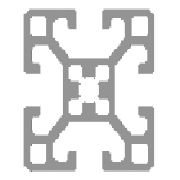
# Autodesk Inventor part: 10-540
Saved by Autodesk Inventor 2022 (Build 260153000, 153)
## iProperties
Created: 2021-12-28
Part Number: 10-540
Material: Generico
Document SubType Name: Modeling
Designer: matte
Standards Organization: 40 series
Language: it-IT
Size Designation: 10-540
Categories: <MemberInstance><Categories><Category DisplayName="Forme strutturali" InternalName="089c4875-fa83-4c05-b084-43b9cc11f5ed" Mnemonic="GRDR"><CategoryParameter DisplayName="Massa per unità di lunghezza" InternalName="0bb95a10-148f-4027-a459-38d7b056702a" Mnemonic="shpmass"/><CategoryParameter DisplayName="Area sezione" InternalName="1ff91680-64b0-4202-b9a3-7fd3f94bba3b" Mnemonic="secarea"/><CategoryParameter DisplayName="Raggio di girazione (x)" InternalName="25778675-03e9-40c1-b6a8-4a9ed693320d" Mnemonic="gyrradx"/><CategoryParameter DisplayName="Modulo di rigidità torsionale" InternalName="26c1ec35-5026-4c63-ad0a-751cf684a536" Mnemonic="torrigmod"/><CategoryParameter DisplayName="Distanza del baricentro X-X" InternalName="26c9bdb8-9c79-4b4f-a92e-8e197583c9c4" Mnemonic="grcendistX"/><CategoryParameter DisplayName="ID membro precedente" InternalName="340afe4f-75d7-48d3-ab7d-943f3c3da468" Mnemonic="LegacyMemberID"/><CategoryParameter DisplayName="Lunghezza base" InternalName="42e34263-8f20-4d0e-ad48-bf1385b87c24" Mnemonic="shplen"/><CategoryParameter DisplayName="Momento di inerzia (y)" InternalName="4b9f58ea-bced-460e-81ea-3d29ca5a49e3" Mnemonic="inermomy"/><CategoryParameter DisplayName="Momento di inerzia (x)" InternalName="4cd780bc-73d7-43ac-917a-579e5cbd684d" Mnemonic="inermomx"/><CategoryParameter DisplayName="Punto di base personalizzato" InternalName="4f1d1b73-316d-484b-a3df-9cbabb16eb77" Mnemonic="shpBasePoint"/><CategoryParameter DisplayName="Altezza forma" InternalName="50274e7d-5ac0-4796-92cb-c59e54983c67" Mnemonic="shpheig"/><CategoryParameter DisplayName="Modulo sezione (y)" InternalName="59eaa5e9-d227-48dc-b6c1-6920f96e0f95" Mnemonic="secmody"/><CategoryParameter DisplayName="Designazione sezione" InternalName="5a64d034-428d-49c8-ba32-7619764de20f" Mnemonic="shpdes"/><CategoryParameter DisplayName="Modulo sezione (x)" InternalName="72cfad18-cf51-4ed4-aaa7-c6b224f8419f" Mnemonic="secmodx"/><CategoryParameter DisplayName="Modulo di sezione torsionale" InternalName="7c55a8dc-8844-49f9-a867-cc677b30ec9a" Mnemonic="torsecmod"/><CategoryParameter DisplayName="Larghezza forma" InternalName="7c717d54-a18f-4666-b4d4-573cce22c62c" Mnemonic="shpwdth"/><CategoryParameter DisplayName="Spessore seconda forma" InternalName="9251a8e1-85fd-4e47-af99-afdb762317d9" Mnemonic="shpthick2"/><CategoryParameter DisplayName="Guarnizione piatta creata" InternalName="9c666724-f362-4ea7-ac62-f6a007de5c69" Mnemonic="shpFGAuto"/><CategoryParameter DisplayName="Distanza del baricentro Y-Y" InternalName="bcc4fb17-7af4-436a-8f8c-d0aa3b0248c5" Mnemonic="grcendistY"/><CategoryParameter DisplayName="Raggio di girazione (y)" InternalName="bfa18ebe-1636-4dbe-8d42-b263e0b73184" Mnemonic="gyrrady"/><CategoryParameter DisplayName="Spessore forma" InternalName="d109cf76-8eb4-42fc-9800-4409734adc67" Mnemonic="shpthick"/><CategoryParameter DisplayName="Coefficiente di spostamento taglio" InternalName="de4c90c6-aaa8-468f-a335-6737b311b5d3" Mnemonic="shdispc"/><Category DisplayName="Altro" InternalName="f02205ff-2390-476f-921c-0b3185f88e84" Mnemonic="OTHSHP"><CategoryParameter DisplayName="Momento di inerzia (y)" InternalName="044c654e-f649-48ac-84cc-650a29ae31ca" Mnemonic="inermomy"/><CategoryParameter DisplayName="Spessore forma" InternalName="12b1a788-9233-48fd-a933-2df8ff42b15f" Mnemonic="shpthick"/><CategoryParameter DisplayName="Massa per unità di lunghezza" InternalName="2fd289d6-9394-4d2d-97e6-6659d7d4551d" Mnemonic="shpmass"/><CategoryParameter DisplayName="Raggio di girazione (y)" InternalName="743e1dfe-1bba-408b-b985-cf752b207386" Mnemonic="gyrrady"/><CategoryParameter DisplayName="Modulo sezione (y)" InternalName="88b8bff9-a616-4028-93d5-ed4f79680d13" Mnemonic="secmody"/><CategoryParameter DisplayName="Area sezione" InternalName="c46ecdf8-b6eb-4db9-8b25-30258930c1e3" Mnemonic="secarea"/><CategoryParameter DisplayName="Modulo sezione (x)" InternalName="cac70804-9d39-43bb-be17-56ea1f39a6c2" Mnemonic="secmodx"/><CategoryParameter DisplayName="Momento di inerzia (x)" InternalName="ec6737bc-264f-43ed-b0bd-f6d410c2718d" Mnemonic="inermomx"/><CategoryParameter DisplayName="Raggio di girazione (x)" InternalName="ee72c61e-565e-4fd6-b448-66e1e1abcb7e" Mnemonic="gyrradx"/></Category></Category><Category DisplayName="TipoDati" InternalName="23b78d0f-2648-40c6-8793-ca6db495c9e8" Mnemonic="DATATYPE"><CategoryParameter DisplayName="NomeVisualizzazione" InternalName="05415f3d-3907-474b-a020-eb9d644f4cf3" Mnemonic="DISPLAYNAME"/><CategoryParameter DisplayName="Norme" InternalName="0c0a119c-1e12-4c84-803f-101930972f5e" Mnemonic="STANDARD"/><CategoryParameter DisplayName="Descrizione" InternalName="13903e3d-64b1-4950-80da-f627842ea37f" Mnemonic="DESCRIPTION"/><CategoryParameter DisplayName="Designazione" InternalName="2675968c-4ce5-49e0-a4f5-552d29089031" Mnemonic="DESIGNATION"/><CategoryParameter DisplayName="Riga di default" InternalName="2af9ec52-faaa-4026-b378-f9fa4afca842" Mnemonic="DEFAULTROW"/><CategoryParameter DisplayName="Nome cartella" InternalName="3f06958e-8713-4116-9be7-ed6184ecc97b" Mnemonic="FOLDERNAME"/><CategoryParameter DisplayName="Guid revisione" InternalName="45a75005-10b1-4dfc-8d6d-dfe629f0b93c" Mnemonic="REVISIONGUID"/><CategoryParameter DisplayName="NomeFile" InternalName="8b46a4cc-9585-4fed-90c3-899f57e09a73" Mnemonic="FILENAME"/><CategoryParameter DisplayName="SocietàNorme" InternalName="8f5914e1-4693-403f-8ab5-d37768198c9d" Mnemonic="STDSORG"/><CategoryParameter DisplayName="Versione famiglia" InternalName="914462f6-6e19-4b14-ba84-155b9680b1d0" Mnemonic="FAMILYREVISION"/><CategoryParameter DisplayName="Revisione norme" InternalName="91d5a463-65c2-4fde-b823-3b7fea5e8e17" Mnemonic="STANDARDREVISION"/><CategoryParameter DisplayName="Revisione membro" InternalName="a65d44b9-392f-4f4f-857b-e4b3d54996fe" Mnemonic="MEMBERREVISION"/><CategoryParameter DisplayName="FormatoPianoRitaglio" InternalName="bc51e27b-3422-4e78-93ef-cec197ddf230" Mnemonic="CLIPFORMAT"/><CategoryParameter DisplayName="Produttore" InternalName="cd6c7a72-a28a-4e50-99a9-2c7f4e13e5ad" Mnemonic="MANUFACTURER"/><CategoryParameter DisplayName="NomeInterno" InternalName="cf1d0246-76d9-4b4a-8305-fa0409afb5c1" Mnemonic="INTERNALNAME"/><CategoryParameter DisplayName="Èmetrico" InternalName="e2385c5b-1ea4-4823-96a8-8de651266ec3" Mnemonic="ISMETRIC"/><Category DisplayName="Parte" InternalName="c0e0b642-3bcb-4cc8-9e80-f96d35c4afa4" Mnemonic="PART"><CategoryParameter DisplayName="Numero parte" InternalName="016b6077-bfbe-49bd-92c9-d8d59c39c941" Mnemonic="PARTNUMBER"/><CategoryParameter DisplayName="Numero di magazzino" InternalName="4dba7c1c-e26c-444e-836c-b08b433409a8" Mnemonic="STOCKNUMBER"/><CategoryParameter DisplayName="Chiave materiale" InternalName="5c9a8adb-dd2b-4535-b97f-0a94a95fe41f" Mnemonic="MATERIALKEY"/><CategoryParameter DisplayName="Materiale" InternalName="818a152a-d3c3-49ca-80ee-df7d91421b8e" Mnemonic="MATERIAL"/></Category></Category></Categories><FamilyTemplate Id="10-540"><FamilyTemplateParameters><FamilyTemplateParameter ObjectType="kModelParameterObject" ValueType="xs:double" Id="12" ObjectReferenceKey="d0"/><FamilyTemplateParameter ObjectType="kPartComponentDefinitionObject" ValueType="xs:string" Id="23" SubObjectId="Material"/><FamilyTemplateParameter ObjectType="kPropertyObject" ValueType="xs:string" Id="26" ObjectReferenceKey="{32853F0F-3444-11d1-9E93-0060B03C1CA6}" SubObjectId="5"/><FamilyTemplateParameter ObjectType="kPropertyObject" ValueType="xs:string" Id="27" ObjectReferenceKey="{32853F0F-3444-11d1-9E93-0060B03C1CA6}" SubObjectId="52"/></FamilyTemplateParameters></FamilyTemplate><CategoryParameterMap><ParamToTemplateMap><ParamToTemplate CategoryParameter="//CategoryParameter[@InternalName='cf1d0246-76d9-4b4a-8305-fa0409afb5c1']" ConstantValue="7d6ce073-411f-4b6a-829f-d390fd53fc07"/><ParamToTemplate CategoryParameter="//CategoryParameter[@InternalName='45a75005-10b1-4dfc-8d6d-dfe629f0b93c']" ConstantValue="1b59e780-9fa2-4ac4-888e-f8f724c6c2fd"/><ParamToTemplate CategoryParameter="//CategoryParameter[@InternalName='3f06958e-8713-4116-9be7-ed6184ecc97b']" ConstantValue="10-540"/><ParamToTemplate CategoryParameter="//CategoryParameter[@InternalName='8f5914e1-4693-403f-8ab5-d37768198c9d']" ConstantValue="40 series"/><ParamToTemplate CategoryParameter="//CategoryParameter[@InternalName='0c0a119c-1e12-4c84-803f-101930972f5e']" TemplateParameter="18"/><ParamToTemplate CategoryParameter="//CategoryParameter[@InternalName='91d5a463-65c2-4fde-b823-3b7fea5e8e17']" TemplateParameter="19"/><ParamToTemplate CategoryParameter="//CategoryParameter[@InternalName='cd6c7a72-a28a-4e50-99a9-2c7f4e13e5ad']" TemplateParameter="20"/><ParamToTemplate CategoryParameter="//CategoryParameter[@InternalName='13903e3d-64b1-4950-80da-f627842ea37f']" TemplateParameter="22"/><ParamToTemplate CategoryParameter="//CategoryParameter[@InternalName='05415f3d-3907-474b-a020-eb9d644f4cf3']" ConstantValue="10-540"/><ParamToTemplate CategoryParameter="//CategoryParameter[@InternalName='914462f6-6e19-4b14-ba84-155b9680b1d0']" ConstantValue="11"/><ParamToTemplate CategoryParameter="//CategoryParameter[@InternalName='bc51e27b-3422-4e78-93ef-cec197ddf230']" ConstantValue="CF_INVENTOR.STDPARTS"/><ParamToTemplate CategoryParameter="//CategoryParameter[@InternalName='e2385c5b-1ea4-4823-96a8-8de651266ec3']" ConstantValue="true"/><ParamToTemplate CategoryParameter="//CategoryParameter[@InternalName='2af9ec52-faaa-4026-b378-f9fa4afca842']" ConstantValue="1"/><ParamToTemplate CategoryParameter="//CategoryParameter[@InternalName='9c666724-f362-4ea7-ac62-f6a007de5c69']" ConstantValue="1"/><ParamToTemplate CategoryParameter="//CategoryParameter[@InternalName='8b46a4cc-9585-4fed-90c3-899f57e09a73']" ConstantValue="10-540"/><ParamToTemplate CategoryParameter="//CategoryParameter[@InternalName='a65d44b9-392f-4f4f-857b-e4b3d54996fe']" ConstantValue="cf6cafbf-75ec-4cf3-9738-ab9345264871"/><ParamToTemplate CategoryParameter="//CategoryParameter[@InternalName='a65d44b9-392f-4f4f-857b-e4b3d54996fe']" ConstantValue="cf6cafbf-75ec-4cf3-9738-ab9345264871"/><ParamToTemplate CategoryParameter="//CategoryParameter[@InternalName='2675968c-4ce5-49e0-a4f5-552d29089031']" TemplateParameter="27"/><ParamToTemplate CategoryParameter="//CategoryParameter[@InternalName='818a152a-d3c3-49ca-80ee-df7d91421b8e']" TemplateParameter="23"/><ParamToTemplate CategoryParameter="//CategoryParameter[@InternalName='016b6077-bfbe-49bd-92c9-d8d59c39c941']" TemplateParameter="26"/><ParamToTemplate CategoryParameter="//CategoryParameter[@InternalName='42e34263-8f20-4d0e-ad48-bf1385b87c24']" TemplateParameter="12"/></ParamToTemplateMap></CategoryParameterMap></MemberInstance>
Density: 1 g/cm^3
Appearance: Default
IsCustomPart: 1
Author: matte
MXEDIT: true
G_L: 100.000 mm
Autodesk Inventor part; units mm, degrees
ref_plane "YZ Plane" through (0, 0, 0) normal (1, 0, 0) x (0, 1, 0)
ref_plane "XY Plane" through (0, 0, 0) normal (0, 0, 1) x (1, 0, 0)
ref_plane "Start Plane" through (0, 0, 0) normal (0, 1, 0) x (-1, 0, 0)
ref_plane "End Plane" through (0, 100, 0) normal (0, 1, 0) x (-1, 0, 0)
sketch "Sketch1" plane through (0, 0, 0) normal (0, 1, 0) x (-1, 0, 0)
  arc A0 (-2.032, 3.5877) -> (-1.3254, 3.1202) centre (-1.524, 3.5877) ccw
  arc A1 (1.3254, 3.1202) -> (-1.3254, 3.1202) centre (0, 0) ccw
  arc A2 (1.3254, 3.1202) -> (2.032, 3.5877) centre (1.524, 3.5877) ccw
  line L0 (2.032, 3.5877) -> (2.032, 5.522)
  arc A3 (2.794, 6.284) -> (2.032, 5.522) centre (2.794, 5.522) ccw
  line L1 (2.794, 6.284) -> (5.522, 6.284)
  arc A4 (6.284, 5.522) -> (5.522, 6.284) centre (5.522, 5.522) ccw
  line L2 (6.284, 5.522) -> (6.284, 2.794)
  arc A5 (5.522, 2.032) -> (6.284, 2.794) centre (5.522, 2.794) ccw
  line L3 (5.522, 2.032) -> (3.5877, 2.032)
  arc A6 (3.5877, 2.032) -> (3.1202, 1.3254) centre (3.5877, 1.524) ccw
  arc A7 (3.1202, -1.3254) -> (3.1202, 1.3254) centre (0, 0) ccw
  arc A8 (3.1202, -1.3254) -> (3.5877, -2.032) centre (3.5877, -1.524) ccw
  line L4 (3.5877, -2.032) -> (5.522, -2.032)
  arc A9 (6.284, -2.794) -> (5.522, -2.032) centre (5.522, -2.794) ccw
  line L5 (6.284, -2.794) -> (6.284, -5.522)
  arc A10 (5.522, -6.284) -> (6.284, -5.522) centre (5.522, -5.522) ccw
  line L6 (5.522, -6.284) -> (2.794, -6.284)
  arc A11 (2.032, -5.522) -> (2.794, -6.284) centre (2.794, -5.522) ccw
  line L7 (2.032, -5.522) -> (2.032, -3.5877)
  arc A12 (2.032, -3.5877) -> (1.3254, -3.1202) centre (1.524, -3.5877) ccw
  arc A13 (-1.3254, -3.1202) -> (1.3254, -3.1202) centre (0, 0) ccw
  arc A14 (-1.3254, -3.1202) -> (-2.032, -3.5877) centre (-1.524, -3.5877) ccw
  line L8 (-2.032, -3.5877) -> (-2.032, -5.522)
  arc A15 (-2.794, -6.284) -> (-2.032, -5.522) centre (-2.794, -5.522) ccw
  line L9 (-2.794, -6.284) -> (-5.522, -6.284)
  arc A16 (-6.284, -5.522) -> (-5.522, -6.284) centre (-5.522, -5.522) ccw
  line L10 (-6.284, -5.522) -> (-6.284, -2.794)
  arc A17 (-5.522, -2.032) -> (-6.284, -2.794) centre (-5.522, -2.794) ccw
  line L11 (-5.522, -2.032) -> (-3.5877, -2.032)
  arc A18 (-3.5877, -2.032) -> (-3.1202, -1.3254) centre (-3.5877, -1.524) ccw
  arc A19 (-3.1202, 1.3254) -> (-3.1202, -1.3254) centre (0, 0) ccw
  arc A20 (-3.1202, 1.3254) -> (-3.5877, 2.032) centre (-3.5877, 1.524) ccw
  line L12 (-3.5877, 2.032) -> (-5.522, 2.032)
  arc A21 (-6.284, 2.794) -> (-5.522, 2.032) centre (-5.522, 2.794) ccw
  line L13 (-6.284, 2.794) -> (-6.284, 5.522)
  arc A22 (-5.522, 6.284) -> (-6.284, 5.522) centre (-5.522, 5.522) ccw
  line L14 (-5.522, 6.284) -> (-2.794, 6.284)
  arc A23 (-2.032, 5.522) -> (-2.794, 6.284) centre (-2.794, 5.522) ccw
  line L15 (-2.032, 5.522) -> (-2.032, 3.5877)
  line L16 (18.4252, 17.1552) -> (18.4252, 14.1732)
  arc A24 (17.1552, 12.9032) -> (18.4252, 14.1732) centre (17.1552, 14.1732) ccw
  line L17 (17.1552, 12.9032) -> (14.1732, 12.9032)
  arc A25 (12.9032, 14.1732) -> (14.1732, 12.9032) centre (14.1732, 14.1732) ccw
  line L18 (12.9032, 14.1732) -> (12.9032, 17.1552)
  arc A26 (14.1732, 18.4252) -> (12.9032, 17.1552) centre (14.1732, 17.1552) ccw
  line L19 (14.1732, 18.4252) -> (17.1552, 18.4252)
  arc A27 (18.4252, 17.1552) -> (17.1552, 18.4252) centre (17.1552, 17.1552) ccw
  line L20 (17.1552, -18.4252) -> (14.1732, -18.4252)
  arc A28 (12.9032, -17.1552) -> (14.1732, -18.4252) centre (14.1732, -17.1552) ccw
  line L21 (12.9032, -17.1552) -> (12.9032, -14.1732)
  arc A29 (14.1732, -12.9032) -> (12.9032, -14.1732) centre (14.1732, -14.1732) ccw
  line L22 (14.1732, -12.9032) -> (17.1552, -12.9032)
  arc A30 (18.4252, -14.1732) -> (17.1552, -12.9032) centre (17.1552, -14.1732) ccw
  line L23 (18.4252, -14.1732) -> (18.4252, -17.1552)
  arc A31 (17.1552, -18.4252) -> (18.4252, -17.1552) centre (17.1552, -17.1552) ccw
  line L24 (-18.4252, -17.1552) -> (-18.4252, -14.1732)
  arc A32 (-17.1552, -12.9032) -> (-18.4252, -14.1732) centre (-17.1552, -14.1732) ccw
  line L25 (-17.1552, -12.9032) -> (-14.1732, -12.9032)
  arc A33 (-12.9032, -14.1732) -> (-14.1732, -12.9032) centre (-14.1732, -14.1732) ccw
  line L26 (-12.9032, -14.1732) -> (-12.9032, -17.1552)
  arc A34 (-14.1732, -18.4252) -> (-12.9032, -17.1552) centre (-14.1732, -17.1552) ccw
  line L27 (-14.1732, -18.4252) -> (-17.1552, -18.4252)
  arc A35 (-18.4252, -17.1552) -> (-17.1552, -18.4252) centre (-17.1552, -17.1552) ccw
  line L28 (-14.1732, 12.9032) -> (-17.1552, 12.9032)
  arc A36 (-18.4252, 14.1732) -> (-17.1552, 12.9032) centre (-17.1552, 14.1732) ccw
  line L29 (-18.4252, 14.1732) -> (-18.4252, 17.1552)
  arc A37 (-17.1552, 18.4252) -> (-18.4252, 17.1552) centre (-17.1552, 17.1552) ccw
  line L30 (-17.1552, 18.4252) -> (-14.1732, 18.4252)
  arc A38 (-12.9032, 17.1552) -> (-14.1732, 18.4252) centre (-14.1732, 17.1552) ccw
  line L31 (-12.9032, 17.1552) -> (-12.9032, 14.1732)
  arc A39 (-14.1732, 12.9032) -> (-12.9032, 14.1732) centre (-14.1732, 14.1732) ccw
  arc A40 (20, 17) -> (17, 20) centre (17, 17) ccw
  line L32 (4.1, 18.5014) -> (4.1, 16.0122)
  arc A41 (4.1, 16.0122) -> (4.608, 15.5042) centre (4.608, 16.0122) ccw
  line L33 (4.608, 15.5042) -> (5.8018, 15.5042)
  arc A42 (5.8018, 15.5042) -> (6.3098, 16.0122) centre (5.8018, 16.0122) ccw
  line L34 (6.3098, 16.0122) -> (6.3098, 17.2822)
  arc A43 (6.8178, 17.7902) -> (6.3098, 17.2822) centre (6.8178, 17.2822) ccw
  line L35 (6.8178, 17.7902) -> (9.9314, 17.7902)
  arc A44 (11.43, 16.2916) -> (9.9314, 17.7902) centre (9.9314, 16.2916) ccw
  line L36 (11.43, 16.2916) -> (11.43, 13.6133)
  arc A45 (10.9911, 12.5536) -> (11.43, 13.6133) centre (9.9314, 13.6133) ccw
  line L37 (10.9911, 12.5536) -> (6.6336, 8.1961)
  arc A46 (5.5739, 7.7572) -> (6.6336, 8.1961) centre (5.5739, 9.2558) ccw
  line L38 (5.5739, 7.7572) -> (-5.5739, 7.7572)
  arc A47 (-6.6336, 8.1961) -> (-5.5739, 7.7572) centre (-5.5739, 9.2558) ccw
  line L39 (-6.6336, 8.1961) -> (-10.9911, 12.5536)
  arc A48 (-11.43, 13.6133) -> (-10.9911, 12.5536) centre (-9.9314, 13.6133) ccw
  line L40 (-11.43, 13.6133) -> (-11.43, 16.2916)
  arc A49 (-9.9314, 17.7902) -> (-11.43, 16.2916) centre (-9.9314, 16.2916) ccw
  line L41 (-9.9314, 17.7902) -> (-6.8178, 17.7902)
  arc A50 (-6.3098, 17.2822) -> (-6.8178, 17.7902) centre (-6.8178, 17.2822) ccw
  line L42 (-6.3098, 17.2822) -> (-6.3098, 16.0122)
  arc A51 (-6.3098, 16.0122) -> (-5.8018, 15.5042) centre (-5.8018, 16.0122) ccw
  line L43 (-5.8018, 15.5042) -> (-4.608, 15.5042)
  arc A52 (-4.608, 15.5042) -> (-4.1, 16.0122) centre (-4.608, 16.0122) ccw
  line L44 (-4.1, 16.0122) -> (-4.1, 18.5014)
  line L45 (-15.5702, 20) -> (-17, 20)
  arc A53 (-17, 20) -> (-20, 17) centre (-17, 17) ccw
  line L46 (-20, 17) -> (-20, 15.5702)
  line L47 (-18.5014, 4.1) -> (-16.0122, 4.1)
  arc A54 (-16.0122, 4.1) -> (-15.5042, 4.608) centre (-16.0122, 4.608) ccw
  line L48 (-15.5042, 4.608) -> (-15.5042, 5.8018)
  arc A55 (-15.5042, 5.8018) -> (-16.0122, 6.3098) centre (-16.0122, 5.8018) ccw
  line L49 (-16.0122, 6.3098) -> (-17.2822, 6.3098)
  arc A56 (-17.7902, 6.8178) -> (-17.2822, 6.3098) centre (-17.2822, 6.8178) ccw
  line L50 (-17.7902, 6.8178) -> (-17.7902, 9.9314)
  arc A57 (-16.2916, 11.43) -> (-17.7902, 9.9314) centre (-16.2916, 9.9314) ccw
  line L51 (-16.2916, 11.43) -> (-13.6133, 11.43)
  arc A58 (-12.5536, 10.9911) -> (-13.6133, 11.43) centre (-13.6133, 9.9314) ccw
  line L52 (-12.5536, 10.9911) -> (-8.1961, 6.6336)
  arc A59 (-7.7572, 5.5739) -> (-8.1961, 6.6336) centre (-9.2558, 5.5739) ccw
  line L53 (-7.7572, 5.5739) -> (-7.7572, -5.5739)
  arc A60 (-8.1961, -6.6336) -> (-7.7572, -5.5739) centre (-9.2558, -5.5739) ccw
  line L54 (-8.1961, -6.6336) -> (-12.5536, -10.9911)
  arc A61 (-13.6133, -11.43) -> (-12.5536, -10.9911) centre (-13.6133, -9.9314) ccw
  line L55 (-13.6133, -11.43) -> (-16.2916, -11.43)
  arc A62 (-17.7902, -9.9314) -> (-16.2916, -11.43) centre (-16.2916, -9.9314) ccw
  line L56 (-17.7902, -9.9314) -> (-17.7902, -6.8178)
  arc A63 (-17.2822, -6.3098) -> (-17.7902, -6.8178) centre (-17.2822, -6.8178) ccw
  line L57 (-17.2822, -6.3098) -> (-16.0122, -6.3098)
  arc A64 (-16.0122, -6.3098) -> (-15.5042, -5.8018) centre (-16.0122, -5.8018) ccw
  line L58 (-15.5042, -5.8018) -> (-15.5042, -4.608)
  arc A65 (-15.5042, -4.608) -> (-16.0122, -4.1) centre (-16.0122, -4.608) ccw
  line L59 (-16.0122, -4.1) -> (-18.5014, -4.1)
  arc A66 (-18.5014, -4.1) -> (-20, -5.5986) centre (-18.5014, -5.5986) ccw
  arc A67 (-20, -17) -> (-17, -20) centre (-17, -17) ccw
  line L60 (-4.1, -18.5014) -> (-4.1, -16.0122)
  arc A68 (-5.5986, -20) -> (-4.1, -18.5014) centre (-5.5986, -18.5014) ccw
  arc A69 (-4.1, -16.0122) -> (-4.608, -15.5042) centre (-4.608, -16.0122) ccw
  line L61 (-4.608, -15.5042) -> (-5.8018, -15.5042)
  arc A70 (-5.8018, -15.5042) -> (-6.3098, -16.0122) centre (-5.8018, -16.0122) ccw
  line L62 (-6.3098, -16.0122) -> (-6.3098, -17.2822)
  arc A71 (-6.8178, -17.7902) -> (-6.3098, -17.2822) centre (-6.8178, -17.2822) ccw
  line L63 (-6.8178, -17.7902) -> (-9.9314, -17.7902)
  arc A72 (-11.43, -16.2916) -> (-9.9314, -17.7902) centre (-9.9314, -16.2916) ccw
  line L64 (-11.43, -16.2916) -> (-11.43, -13.6133)
  arc A73 (-10.9911, -12.5536) -> (-11.43, -13.6133) centre (-9.9314, -13.6133) ccw
  line L65 (-10.9911, -12.5536) -> (-6.6336, -8.1961)
  arc A74 (-5.5739, -7.7572) -> (-6.6336, -8.1961) centre (-5.5739, -9.2558) ccw
  line L66 (-5.5739, -7.7572) -> (5.5739, -7.7572)
  arc A75 (6.6336, -8.1961) -> (5.5739, -7.7572) centre (5.5739, -9.2558) ccw
  line L67 (6.6336, -8.1961) -> (10.9911, -12.5536)
  arc A76 (11.43, -13.6133) -> (10.9911, -12.5536) centre (9.9314, -13.6133) ccw
  line L68 (11.43, -13.6133) -> (11.43, -16.2916)
  arc A77 (9.9314, -17.7902) -> (11.43, -16.2916) centre (9.9314, -16.2916) ccw
  line L69 (9.9314, -17.7902) -> (6.8178, -17.7902)
  arc A78 (6.3098, -17.2822) -> (6.8178, -17.7902) centre (6.8178, -17.2822) ccw
  line L70 (6.3098, -17.2822) -> (6.3098, -16.0122)
  arc A79 (6.3098, -16.0122) -> (5.8018, -15.5042) centre (5.8018, -16.0122) ccw
  line L71 (5.8018, -15.5042) -> (4.608, -15.5042)
  arc A80 (4.608, -15.5042) -> (4.1, -16.0122) centre (4.608, -16.0122) ccw
  line L72 (4.1, -16.0122) -> (4.1, -18.5014)
  arc A81 (4.1, -18.5014) -> (5.5986, -20) centre (5.5986, -18.5014) ccw
  arc A82 (17, -20) -> (20, -17) centre (17, -17) ccw
  line L73 (18.5014, -4.1) -> (16.0122, -4.1)
  arc A83 (20, -5.5986) -> (18.5014, -4.1) centre (18.5014, -5.5986) ccw
  arc A84 (16.0122, -4.1) -> (15.5042, -4.608) centre (16.0122, -4.608) ccw
  line L74 (15.5042, -4.608) -> (15.5042, -5.8018)
  arc A85 (15.5042, -5.8018) -> (16.0122, -6.3098) centre (16.0122, -5.8018) ccw
  line L75 (16.0122, -6.3098) -> (17.2822, -6.3098)
  arc A86 (17.7902, -6.8178) -> (17.2822, -6.3098) centre (17.2822, -6.8178) ccw
  line L76 (17.7902, -6.8178) -> (17.7902, -9.9314)
  arc A87 (16.2916, -11.43) -> (17.7902, -9.9314) centre (16.2916, -9.9314) ccw
  line L77 (16.2916, -11.43) -> (13.6133, -11.43)
  arc A88 (12.5536, -10.9911) -> (13.6133, -11.43) centre (13.6133, -9.9314) ccw
  line L78 (12.5536, -10.9911) -> (8.1961, -6.6336)
  arc A89 (7.7572, -5.5739) -> (8.1961, -6.6336) centre (9.2558, -5.5739) ccw
  line L79 (7.7572, -5.5739) -> (7.7572, 5.5739)
  arc A90 (8.1961, 6.6336) -> (7.7572, 5.5739) centre (9.2558, 5.5739) ccw
  line L80 (8.1961, 6.6336) -> (12.5536, 10.9911)
  arc A91 (13.6133, 11.43) -> (12.5536, 10.9911) centre (13.6133, 9.9314) ccw
  line L81 (13.6133, 11.43) -> (16.2916, 11.43)
  arc A92 (17.7902, 9.9314) -> (16.2916, 11.43) centre (16.2916, 9.9314) ccw
  line L82 (17.7902, 9.9314) -> (17.7902, 6.8178)
  arc A93 (17.2822, 6.3098) -> (17.7902, 6.8178) centre (17.2822, 6.8178) ccw
  line L83 (17.2822, 6.3098) -> (16.0122, 6.3098)
  arc A94 (16.0122, 6.3098) -> (15.5042, 5.8018) centre (16.0122, 5.8018) ccw
  line L84 (15.5042, 5.8018) -> (15.5042, 4.608)
  arc A95 (15.5042, 4.608) -> (16.0122, 4.1) centre (16.0122, 4.608) ccw
  line L85 (16.0122, 4.1) -> (18.5014, 4.1)
  line L86 (-15.5702, 20) -> (-5.5986, 20)
  arc A96 (-4.1, 18.5014) -> (-5.5986, 20) centre (-5.5986, 18.5014) ccw
  line L87 (-20, 15.5702) -> (-20, 5.5986)
  arc A97 (-20, 5.5986) -> (-18.5014, 4.1) centre (-18.5014, 5.5986) ccw
  line L88 (17, 20) -> (5.5986, 20)
  arc A98 (5.5986, 20) -> (4.1, 18.5014) centre (5.5986, 18.5014) ccw
  line L89 (20, 17) -> (20, 5.5986)
  arc A99 (18.5014, 4.1) -> (20, 5.5986) centre (18.5014, 5.5986) ccw
  line L90 (20, -17) -> (20, -5.5986)
  line L91 (17, -20) -> (5.5986, -20)
  line L92 (-17, -20) -> (-5.5986, -20)
  line L93 (-20, -17) -> (-20, -5.5986)
  constraints: 200 point on circle, 188 end point, 100 centre point, 43 horizontal, 43 vertical, 403 other
extrude "Body" add sketch "Sketch1" along normal up to surface (100 mm away) from surface at 0
sketch "Sketch2" plane through (0, 0, 0) normal (0, 1, 0) x (-1, 0, 0)
  line L0 (0, 0) -> (10, 0)
ref_plane "Work Plane3" through (0, 0, 0) normal (0, 0, -1) x (-1, 0, 0)
sketch "Sketch3" plane through (0, 0, 0) normal (0, 0, -1) x (-1, 0, 0)
  line L0 (-28, 0) -> (28, 0)
  line L1 (-28, 100) -> (28, 100)
  dimension "d7" = 100
  measures "d7" distance between parallel lines of L0 L1
equation "\"G_OFFSET_START\" = 0"
equation "\"G_OFFSET_END\" = 0"
equation "\"G_L\" = d7"
body "Solid1"
